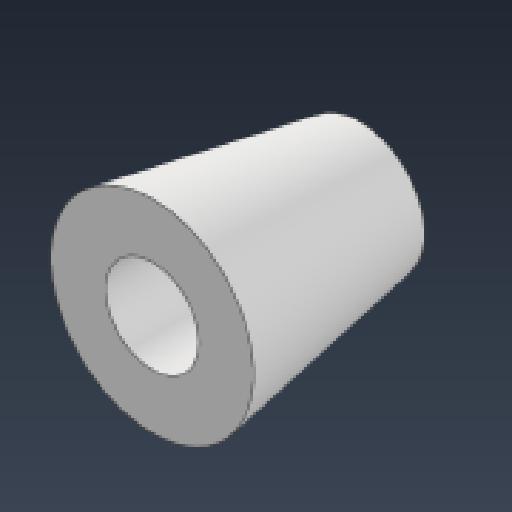
# Autodesk Inventor part: hold-fur-wylewanko
Saved by Autodesk Inventor 2023 (Build 270158000, 158)
## iProperties
Created: 2025-10-29
Part Number: hold-fur-wylewanko
Material: Generic
Document SubType Name: Modeling
Designer: szymo
Density: 1 g/cm^3
Appearance: Default
Author: szymo
Autodesk Inventor part; units mm, degrees
ref_plane "YZ Plane" through (0, 0, 0) normal (1, 0, 0) x (0, 1, 0)
ref_plane "XZ Plane" through (0, 0, 0) normal (0, 1, 0) x (-1, 0, 0)
ref_plane "XY Plane" through (0, 0, 0) normal (0, 0, 1) x (1, 0, 0)
sketch "Sketch1" plane through (0, 0, 0) normal (1, 0, 0) x (0, 1, 0)
  line L0 (3.5, -0.5) -> (10.1, -0.5) projected
  line L1 (6.8, -0.5) -> (6.8, -5.5)
  line L2 (2.8894, 2.5) -> (6.8, 2.5)
  line L3 (6.8, 2.5) -> (6.8, -0.5)
  line L4 (6.8, -5.5) -> (4.3, -5.5)
  line L5 (4.3, -5.5) -> (2.8894, 2.5)
  point P0 (0, 0)
  dimension "d0" = 3.3
  dimension "d1" = 3.3
  dimension "d2" = 2.5
  dimension "d3" = 5
  dimension "d4" = 3
  dimension "d5" = 80
  constraints: 10 end point, 2 perpendicular, 1 horizontal, 1 midpoint, 1 point on line, 1 vertical
  measures "d0" distance of L0.end L1.start
  measures "d1" distance of L0.start L1.start
  measures "d2" distance of L1.end L4.end
  measures "d3" distance between parallel lines of L4 L0
  measures "d4" distance between parallel lines of L2 L0
  measures "d5" angle of L2 L5
revolve "Revolution1" add sketch "Sketch1" angle 360 about axis through (0, 6.8, 2.5) along (0, 0, -1)
sketch "Sketch2" plane through (0, 6.8, 2.5) normal (0, 0, 1) x (1, 0, 0)
  circle A0 centre (0, 0) radius 3.9106 projected
  point P0 (0, -6.8)
  constraints: 1 coincident
hole "Hole1" at (0, 6.8, 2.5) direction (0, 0, -1) diameter 3.6 depth 8.8 clearance for "Countersunk Flat Head Screw ISO 2009/7046" size "M3" standard "ISO"
body "Solid1"
